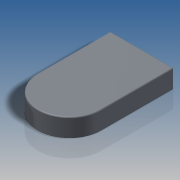
# Autodesk Inventor part: 76610-LtBluishGray
Saved by Autodesk Inventor 2016 SP2 (Build 200236200, 236)
## iProperties
Created: 2015-08-26
Part Number: 76610-LtBluishGray
Material: ABS Plastic
Document SubType Name: Modeling
Designer: D. Kohfeld
Mass: 0.0816023 g
Surface Area: 1.3851 cm^2
Volume: 0.0769833 cm^3
Density: 1.06 g/cm^3
Appearance: LtBluishGray
Author: D. Kohfeld
Autodesk Inventor part; units mm, degrees
ref_plane "YZ Plane" through (0, 0, 0) normal (1, 0, 0) x (0, 1, 0)
ref_plane "XZ Plane" through (0, 0, 0) normal (0, 1, 0) x (-1, 0, 0)
ref_plane "XY Plane" through (0, 0, 0) normal (0, 0, 1) x (1, 0, 0)
sketch "Sketch2" plane through (0, 0, 0) normal (0, 1, 0) x (-1, 0, 0)
  line L0 (-2.8, -6.4) -> (2.8, -6.4)
  line L1 (2.8, -6.4) -> (2.8, 0)
  arc A0 (2.8, 0) -> (-2.8, 0) centre (0, 0) ccw
  line L2 (-2.8, 0) -> (-2.8, -6.4)
  dimension "d0" = 6.4
  dimension "d1" = 5.6
  constraints: 6 end point, 2 point on circle, 2 tangent, 2 vertical, 1 centre point, 1 coincident, 1 horizontal
  measures "d0" distance from line of point (0, 0) L0
  measures "d1" distance between parallel lines of L1 L2
extrude "Extrusion1" add sketch "Sketch2" along normal mid plane 1.6
fillet "Fillet1" radius 0.1 6 edges at (0, 0.8, 2.8) (2.8, 0.8, -3.2) (-2.8, 0.8, -3.2) (-2.8, 0, -6.4) (0, 0.8, -6.4) (2.8, 0, -6.4)
equation "\"d2\" = wall"
equation "\"wall\" = 1.6"
body "Solid1"
